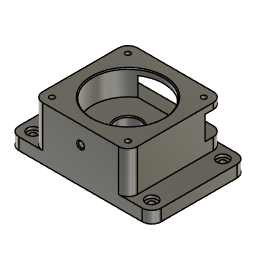
metrology_MODEL (Autodesk Fusion 360 design; units mm, degrees)
Autodesk Fusion 360 part; units mm, degrees
sketch "Sketch1" plane through (0, 0, 0) normal (0, 0, 1) x (1, 0, 0)
  line L0 (3, -2) -> (-3, -2)
  line L1 (-3, -2) -> (-3, 2)
  line L2 (-3, 2) -> (3, 2)
  line L3 (3, 2) -> (3, -2)
  line L4 (3, -2) -> (-3, 2) construction
  line L5 (-3, -2) -> (3, 2) construction
  circle A0 centre (0, 0) radius 1.75
  circle A1 centre (0, 0) radius 1.25
  circle A2 centre (0, 0) radius 0.5
  dimension "d1" = 6
  dimension "d2" = 4
  dimension "d3" = 3.5
  dimension "d4" = 2.5
  dimension "d5" = 1
  constraint horizontal L0
  constraint perpendicular L0 L1
  constraint parallel L0 L2
  constraint parallel L1 L3
  constraint coincident L4 A0.centre
  constraint coincident L5 A0.centre
  constraint coincident A0.centre A1.centre
  constraint concentric A1 A2
  measures "d1" distance of L1.end L2.end
  measures "d2" distance of L0.end L1.end
  measures "d3" diameter of A0
  measures "d4" diameter of A1
  measures "d5" diameter of A2
extrude "Extrude1" add sketch "Sketch1" along normal blind 2.25 contours L0 L1 L2 L3 | A0 | A1 | A2
extrude "Extrude2" cut sketch "Sketch1" along normal blind 0.25 contours A0 | A1 | A2
extrude "Extrude3" cut sketch "Sketch1" along normal blind 0.75 contours A1
extrude "Extrude4" cut sketch "Sketch1" along normal blind 2.7 contours A2
sketch "Sketch2" plane through (0, 0, 2.25) normal (0, 0, 1) x (-1, 0, 0)
  circle A0 centre (0, 0) radius 0.5
  line L0 (-3, -2) -> (3, -2)
  line L1 (3, -2) -> (3, 2)
  line L2 (3, 2) -> (-3, 2)
  line L3 (-3, 2) -> (-3, -2)
  circle A1 centre (0, 0) radius 1.5
  line L4 (2, 2) -> (-2, 2)
  line L5 (-2, 2) -> (-2, -2)
  line L6 (-2, -2) -> (2, -2)
  line L7 (2, -2) -> (2, 2)
  line L8 (2, 2) -> (-2, -2) construction
  line L9 (-2, 2) -> (2, -2) construction
  line L10 (2, -2) -> (1.6, -2)
  line L11 (2, -1.6) -> (2, -2)
  line L12 (-2, -2) -> (-1.6, -2)
  line L13 (-2, -1.6) -> (-2, -2)
  line L14 (2, 1.6) -> (2, 2)
  line L15 (-2, 2) -> (-1.6, 2)
  line L16 (-2, 1.6) -> (-2, 2)
  circle A2 centre (-1.6, 1.6) radius 0.106
  circle A3 centre (1.6, 1.6) radius 0.106
  circle A4 centre (1.6, -1.6) radius 0.106
  circle A5 centre (-1.6, -1.6) radius 0.106
  dimension "d14" = 3
  dimension "d23" = 4
  dimension "d24" = 4
  dimension "d47" = 0.4
  dimension "d48" = 0.4
  dimension "d49" = 0.4
  dimension "d50" = 0.4
  dimension "d52" = 0.4
  dimension "d53" = 0.4
  dimension "d54" = 0.4
  dimension "d55" = 0.212
  dimension "d56" = 0.212
  dimension "d57" = 0.212
  dimension "d58" = 0.212
  constraint coincident A0.centre A1.centre
  constraint horizontal L4
  constraint perpendicular L4 L5
  constraint parallel L4 L6
  constraint parallel L5 L7
  constraint coincident L8 A0.centre
  constraint coincident L9 A0.centre
  constraint horizontal L10
  constraint vertical L11
  constraint horizontal L12
  constraint vertical L13
  constraint vertical L14
  constraint horizontal L15
  constraint vertical L16
  measures "d14" diameter of A1
  measures "d23" distance of L5.end L6.end
  measures "d24" distance of L4.end L5.end
  measures "d47" distance of L6.end L10.end
  measures "d48" distance of L6.end L11.start
  measures "d49" distance of L5.end L12.end
  measures "d50" distance of L5.end L13.start
  measures "d52" distance of L4.start L14.start
  measures "d53" distance of L4.end L15.end
  measures "d54" distance of L4.end L16.start
  measures "d55" diameter of A2
  measures "d56" diameter of A3
  measures "d57" diameter of A4
  measures "d58" diameter of A5
extrude "Extrude5" cut sketch "Sketch2" against normal blind 1.05 contours A1
sketch "Sketch3" plane through (-3, 0, 0) normal (-1, 0, 0) x (0, -1, 0)
  line L0 (-2, 0) -> (2, 0)
  line L1 (2, 0) -> (2, 2.25)
  line L2 (2, 2.25) -> (-2, 2.25)
  line L3 (-2, 2.25) -> (-2, 0)
  line L4 (-2, 0) -> (-2, 1)
  line L5 (-2, 1) -> (-2, 2)
  line L6 (-2, 2) -> (-1.25, 2)
  line L7 (-1.25, 2) -> (-1.25, 1)
  line L8 (-1.25, 1) -> (-2, 1)
  dimension "d17" = 1
  dimension "d18" = 1
  dimension "d19" = 0.75
  dimension "d20" = 1
  constraint coincident L0.start L3.end
  constraint perpendicular L0 L4
  constraint coincident L3 L5.end
  constraint perpendicular L3 L6
  constraint perpendicular L6 L7
  measures "d17" distance of L0.start L4.end
  measures "d18" distance of L4.end L5.end
  measures "d19" distance of L5.end L6.end
  measures "d20" distance of L6.end L7.end
extrude "Extrude6" cut sketch "Sketch3" against normal blind 6.4 contours L3 L5 L6 L7 L8
extrude "Extrude7" cut sketch "Sketch2" against normal blind 1.75 contours L0 L1 L2 L7 L11 L14
extrude "Extrude8" cut sketch "Sketch2" against normal blind 1.75 contours L0 L2 L3 L5 L13 L16
sketch "Sketch4" plane through (0, 0, 0.5) normal (0, 0, 1) x (-1, 0, 0)
  line L0 (-3, 2) -> (-3, -2)
  line L1 (-3, -2) -> (-2, -2)
  line L2 (-2, -2) -> (-2, 2)
  line L3 (-2, 2) -> (-3, 2)
  circle A0 centre (-2.5, -1.5) radius 0.25
  circle A1 centre (-2.5, -1.5) radius 0.125
  circle A2 centre (-2.5, 1.5) radius 0.25
  circle A3 centre (-2.5, 1.5) radius 0.125
  circle A4 centre (2.5, 1.5) radius 0.25
  circle A5 centre (2.5, 1.5) radius 0.125
  circle A6 centre (2.5, -1.5) radius 0.25
  circle A7 centre (2.5, -1.5) radius 0.125
  dimension "d31" = 0.5
  dimension "d32" = 0.25
  constraint concentric A0 A1
  measures "d31" diameter of A0
  measures "d32" diameter of A1
extrude "Extrude9" cut sketch "Sketch4" against normal blind 0.125 contours A0 | A1 | A2 | A3 | A4 | A5 | A6 | A7
extrude "Extrude10" cut sketch "Sketch4" against normal blind 1.3 contours A1 | A3 | A5 | A7
chamfer "Chamfer1" distance 0.04 angle 45 3 edges at (1.3985, -0.5424, 2.25) (-0.4662, -0.1808, 1.2) (-0.4662, 0.1808, 0.75)
chamfer "Chamfer2" distance 0.04 angle 45 2 edges at (-1.6316, -0.6328, 0) (-1.1654, -0.452, 0.25)
fillet "Fillet1" radius 0.4 1 edges at (-3, 2, 0.25)
fillet "Fillet2" radius 0.4 3 edges at (-3, -2, 0.25) (3, -2, 0.25) (3, 2, 0.25)
fillet "Fillet3" radius 0.4 4 edges at (-2, 2, 2.125) (-2, 2, 0.75) (2, 2, 2.125) (2, 2, 0.75)
fillet "Fillet4" radius 0.4 2 edges at (-2, -2, 1.375) (2, -2, 1.375)
extrude "Extrude11" cut sketch "Sketch2" against normal blind 0.8 contours A2 | A3 | A4 | A5
sketch "Sketch5" plane through (0, -2, 0) normal (0, -1, 0) x (1, 0, 0)
  line L0 (2.6, 0.5) -> (1.6, 0.5)
  line L1 (1.6, 0.5) -> (1.6, 2.25)
  line L2 (1.6, 2.25) -> (-1.6, 2.25)
  line L3 (-1.6, 2.25) -> (-1.6, 0.5)
  line L4 (-1.6, 0.5) -> (-2.6, 0.5)
  line L5 (-2.6, 0.5) -> (-2.6, 0)
  line L6 (-2.6, 0) -> (2.6, 0)
  line L7 (2.6, 0) -> (2.6, 0.5)
  circle A0 centre (0, 1.5) radius 0.125
  dimension "d61" = 1.5
  dimension "d62" = 0.25
  measures "d61" distance of origin A0.centre
  measures "d62" diameter of A0
extrude "Extrude12" cut sketch "Sketch5" against normal blind 0.9 contours A0
chamfer "Chamfer3" distance 0.04 angle 45 1 edges at (-0.1165, -2, 1.5452)
